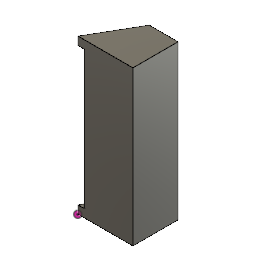
cutter (Autodesk Fusion 360 design; units mm, degrees)
Autodesk Fusion 360 part; units mm, degrees
sketch "Sketch1" plane through (0, 0, 0) normal (0, 1, 0) x (1, 0, 0)
form "Form1" [no effect]
sketch "Sketch2" plane through (0, 0, 0) normal (0, 1, 0) x (1, 0, 0)
  line L0 (0, 0) -> (3.349, -0.0022)
  line L1 (0, 0) -> (9.4772, 16.415)
  line L2 (0, 0) -> (18.954, 0) construction
  line L3 (3.349, -0.0022) -> (20.743, -0.0022) construction
  line L4 (9.217, 15.9643) -> (11.749, 14.5463)
  line L5 (0, 0) -> (9.217, 15.9643)
  line L6 (9.217, 15.9643) -> (10.9491, 14.9643)
  line L7 (10.9491, 14.9643) -> (1.7321, -1)
  line L8 (1.7321, -1) -> (0, 0)
  line L9 (0, 0) -> (20, 0)
  line L10 (20, 0) -> (20, 16.415)
  line L11 (9.4772, 16.415) -> (0, 16.415)
  line L12 (0, 16.415) -> (0, 0)
  line L13 (20, 16.415) -> (9.4772, 16.415)
  line L14 (0, 0) -> (4.25, 7.3612)
  line L15 (4.25, 7.3612) -> (5, 8.6603)
  line L16 (4.25, 7.3612) -> (3.5, 6.0622)
  line L17 (3.5, 6.0622) -> (5, 8.6603)
  dimension "d4" = 3.349
  dimension "d6" = 60
  dimension "d9" = 16.415
  dimension "d10" = 20
  dimension "d23" = 2
  dimension "d24" = 18.434
  measures "d4" distance of L0.start
  measures "d6" angle of L1 L2
  measures "d9" distance of L0.start
  measures "d23" distance of L5 L7
  measures "d24" distance of L0.start
extrude "Extrude3" add sketch "Sketch2" along normal blind 3 contours L0 L1 L5 L6 L7 L9 L14 L15 L16 L17 | L1 L6 L7 L9 L10 L13 makes body 1
extrude "Extrude2" add sketch "Sketch2" along normal blind 53 separate body contours L1 L6 L7 L9 L10 L13 makes body 2
extrude "Extrude1" add sketch "Sketch2" along normal blind 3 separate body contours L0 L1 L5 L6 L7 L9 L14 L15 L16 L17 | L1 L6 L7 L9 L10 L13 makes body 3
move_body "Move1" bodies 3 to x (1, 0, 0) y (0, 1, 0) z (0, 0, 1) at (0, 53, 0)
combine "Combine1" operation add target body 3 tool bodies 2 1
